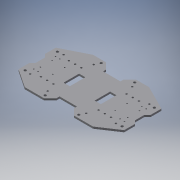
# Autodesk Inventor part: Support_Moteur
Saved by Autodesk Inventor 2016 (Build 200138000, 138)
## iProperties
Created: 2015-09-29
Part Number: Support_Moteur
Material: Générique
Document SubType Name: Modeling
Designer: Logan
Density: 1 g/cm^3
Appearance: Par défaut
Author: Logan
Autodesk Inventor part; units mm, degrees
ref_plane "YZ Plane" through (0, 0, 0) normal (1, 0, 0) x (0, 1, 0)
ref_plane "XZ Plane" through (0, 0, 0) normal (0, 1, 0) x (-1, 0, 0)
ref_plane "XY Plane" through (0, 0, 0) normal (0, 0, 1) x (1, 0, 0)
sketch "Esquisse1" plane through (0, 0, 0) normal (0, 0, 1) x (1, 0, 0)
  line L0 (-170, -60) -> (-170, 60)
  line L1 (170, 60) -> (170, -60)
  line L2 (170, -100) -> (-170, 100) construction
  line L3 (-170, -100) -> (170, 100) construction
  line L4 (-90, 100) -> (-170, 60)
  line L5 (90, 100) -> (170, 60)
  line L6 (-170, -60) -> (-110, -100)
  line L7 (110, -100) -> (170, -60)
  line L8 (48, 100) -> (90, 100)
  line L9 (52, 0) -> (-69, 0)
  line L10 (28, -80) -> (28, -70)
  line L11 (28, -70) -> (-28, -70)
  line L12 (-28, -70) -> (-28, -80)
  line L13 (-28, -80) -> (-48, -100)
  line L14 (28, -80) -> (48, -100)
  line L15 (110, -100) -> (48, -100)
  line L16 (-48, -100) -> (-110, -100)
  line L17 (-28, 70) -> (-28, 80)
  line L18 (-28, 80) -> (-48, 100)
  line L19 (28, 70) -> (-28, 70)
  line L20 (28, 80) -> (28, 70)
  line L21 (28, 80) -> (48, 100)
  line L22 (-90, 100) -> (-48, 100)
  line L23 (48, 100) -> (90, 100)
  point P0 (0, 0)
  dimension "d2" = 80
  dimension "d3" = 40
  dimension "d4" = 80
  dimension "d5" = 40
  dimension "d6" = 40
  dimension "d7" = 60
  dimension "d8" = 60
  dimension "d9" = 40
  constraints: 48 end point, 7 parallel, 6 symmetric about line, 4 point on line, 3 horizontal, 2 collinear, 2 midpoint, 2 perpendicular
  measures "d2" distance of L4.start L2.end
  measures "d3" distance of L0.end L2.end
  measures "d4" distance of L5.start L3.end
  measures "d5" distance of L1.start L3.end
  measures "d6" distance of L0.start L3.start
  measures "d7" distance of L6.end L3.start
  measures "d8" distance of L7.start L2.start
  measures "d9" distance of L1.end L2.start
extrude "Plaque" add sketch "Esquisse1" along normal blind 6
sketch "Esquisse2" plane through (0, 0, 6) normal (0, 0, 1) x (1, 0, 0)
  circle A0 centre (-146, 35) radius 2
  circle A1 centre (-132, 35) radius 2
  circle A2 centre (-146, -35) radius 2
  circle A3 centre (-132, -35) radius 2
  line L0 (-170, 60) -> (-170, -60) projected
  line L1 (0, 25.5561) -> (0, -26.1527)
  circle A4 centre (146, 35) radius 2
  circle A5 centre (132, 35) radius 2
  circle A6 centre (146, -35) radius 2
  circle A7 centre (132, -35) radius 2
  point P0 (0, 0)
  dimension "d12" = 4
  dimension "d13" = 4
  dimension "d14" = 4
  dimension "d15" = 4
  dimension "d16" = 14
  dimension "d17" = 14
  dimension "d18" = 24
  dimension "d19" = 24
  dimension "d20" = 35
  dimension "d21" = 35
  dimension "d22" = 35
  dimension "d23" = 35
  constraints: 8 centre point, 4 symmetric about line, 2 end point, 1 vertical, 4 other
  measures "d12" diameter of A0
  measures "d13" diameter of A1
  measures "d14" diameter of A3
  measures "d15" diameter of A2
  measures "d16" distance of A1.centre A0.centre
  measures "d17" distance of A3.centre A2.centre
  measures "d18" distance from line of L0 A0.centre
  measures "d19" distance from line of L0 A2.centre
  measures "d20" vertical distance of point (0, 0) A2.centre
  measures "d21" vertical distance of point (0, 0) A3.centre
  measures "d22" vertical distance of point (0, 0) A1.centre
  measures "d23" vertical distance of point (0, 0) A0.centre
hole "Fixation_Encodeur" at (-132, 35, 6) at (-146, 35, 6) at (-146, -35, 6) at (-132, -35, 6) at (132, 35, 6) at (146, 35, 6) at (146, -35, 6) at (132, -35, 6) direction (0, 0, -1) diameter 4 end through all
sketch "Esquisse3" plane through (0, 0, 6) normal (0, 0, 1) x (1, 0, 0)
  line L0 (-140.5, -19) -> (-100.5, -19)
  line L1 (-100.5, -19) -> (-100.5, 19)
  line L2 (-100.5, 19) -> (-140.5, 19)
  line L3 (-140.5, 19) -> (-140.5, -19)
  line L4 (-140.5, -19) -> (-100.5, 19) construction
  line L5 (-100.5, -19) -> (-140.5, 19) construction
  line L6 (-90, 100) -> (-170, 60) projected
  line L7 (-170, 60) -> (-170, -60) projected
  line L8 (-170, -60) -> (-110, -100) projected
  line L9 (48, -100) -> (110, -100) projected
  line L10 (110, -100) -> (170, -60) projected
  line L11 (170, -60) -> (170, 60) projected
  line L12 (170, 60) -> (90, 100) projected
  line L13 (-48, 100) -> (-90, 100) projected
  line L14 (0, 102.1518) -> (0, -90)
  line L15 (140.5, -19) -> (100.5, -19)
  line L16 (100.5, -19) -> (100.5, 19)
  line L17 (100.5, 19) -> (140.5, 19)
  line L18 (140.5, 19) -> (140.5, -19)
  line L19 (140.5, -19) -> (100.5, 19) construction
  line L20 (100.5, -19) -> (140.5, 19) construction
  line L21 (-110, -100) -> (-48, -100) projected
  line L22 (-48, -100) -> (-28, -80) projected
  line L23 (-28, -80) -> (-28, -70) projected
  line L24 (-28, -70) -> (28, -70) projected
  line L25 (28, -70) -> (28, -80) projected
  line L26 (28, -80) -> (48, -100) projected
  line L27 (90, 100) -> (48, 100) projected
  line L28 (48, 100) -> (28, 80) projected
  line L29 (28, 80) -> (28, 70) projected
  line L30 (28, 70) -> (-28, 70) projected
  line L31 (-28, 70) -> (-28, 80) projected
  line L32 (-28, 80) -> (-48, 100) projected
  point P0 (0, 0)
  point P1 (-120.5, 0)
  point P2 (120.5, 0)
  dimension "d31" = 29.5
  dimension "d32" = 40
  dimension "d33" = 38
  dimension "d53" = 19
  constraints: 26 end point, 5 symmetric about line, 4 midpoint, 2 parallel, 1 horizontal, 1 perpendicular, 1 vertical
  measures "d31" distance between parallel lines of L7 L3
  measures "d32" distance between parallel lines of L3 L1
  measures "d33" distance between parallel lines of L0 L2
  measures "d53" distance from line of point (0, 0) L2
hole "Fixation_Moteur" at (-140.5, 19, 6) at (-100.5, 19, 6) at (-100.5, -19, 6) at (-140.5, -19, 6) at (140.5, 19, 6) at (140.5, -19, 6) at (100.5, 19, 6) at (100.5, -19, 6) direction (0, 0, -1) diameter 4 end through all
sketch "Esquisse4" plane through (0, 0, 6) normal (0, 0, 1) x (1, 0, 0)
  line L0 (-60, -25) -> (-40, -25)
  line L1 (-60, 25) -> (-60, -25)
  line L2 (-60, -25) -> (-39.915, 7.067) construction
  circle A0 centre (100.5, 19) radius 2 projected
  circle A1 centre (140.5, 19) radius 2 projected
  circle A2 centre (-100.5, -19) radius 2 projected
  circle A3 centre (-140.5, 19) radius 2 projected
  circle A4 centre (-100.5, 19) radius 2 projected
  circle A5 centre (-140.5, -19) radius 2 projected
  circle A6 centre (140.5, -19) radius 2 projected
  circle A7 centre (100.5, -19) radius 2 projected
  line L3 (-90, 100) -> (-170, 60) projected
  line L4 (-170, 60) -> (-170, -60) projected
  line L5 (-170, -60) -> (-110, -100) projected
  line L6 (48, -100) -> (110, -100) projected
  line L7 (110, -100) -> (170, -60) projected
  line L8 (170, -60) -> (170, 60) projected
  line L9 (170, 60) -> (90, 100) projected
  line L10 (-48, 100) -> (-90, 100) projected
  line L11 (40, 25) -> (60, 25)
  line L12 (60, 25) -> (60, -25)
  line L13 (60, -25) -> (40, -10.6364) construction
  line L14 (40, 25) -> (40, -25)
  line L15 (-40, -25) -> (-40, 25)
  line L16 (-40, 25) -> (-60, 25)
  line L17 (-39.915, 7.067) -> (-60, 25) construction
  line L18 (40, 10.0232) -> (60, 25) construction
  line L19 (60, -25) -> (40, -25)
  line L20 (-110, -100) -> (-48, -100) projected
  line L21 (-48, -100) -> (-28, -80) projected
  line L22 (-28, -80) -> (-28, -70) projected
  line L23 (-28, -70) -> (28, -70) projected
  line L24 (28, -70) -> (28, -80) projected
  line L25 (28, -80) -> (48, -100) projected
  line L26 (90, 100) -> (48, 100) projected
  line L27 (48, 100) -> (28, 80) projected
  line L28 (28, 80) -> (28, 70) projected
  line L29 (28, 70) -> (-28, 70) projected
  line L30 (-28, 70) -> (-28, 80) projected
  line L31 (-28, 80) -> (-48, 100) projected
  point P0 (-39.915, 7.067)
  dimension "d50" = 110
  dimension "d157" = 110
  dimension "d158" = 20
  dimension "d159" = 20
  constraints: 24 end point, 3 point on line, 2 collinear, 2 parallel, 1 horizontal
  measures "d50" distance between parallel lines of L4 L1
  measures "d157" distance between parallel lines of L8 L12
  measures "d158" distance between parallel lines of L1 L15
  measures "d159" distance between parallel lines of L12 L14
extrude "Passage_Courroie" cut sketch "Esquisse4" against normal up to surface (6 mm away) contours L1 L16 L15 L0 | L11 L12 L19 L14
sketch "Esquisse5" plane through (0, 0, 6) normal (0, 0, 1) x (1, 0, 0)
  line L0 (0, 30.4597) -> (0, -30.4597)
  line L1 (-17.5456, 0) -> (17.5456, 0)
  line L2 (-80, 40) -> (-80, -40)
  line L3 (-80, -40) -> (-110, -40)
  line L4 (-110, 30) -> (-110, 40)
  line L5 (-110, 40) -> (-80, 40)
  line L6 (-88, 90) -> (-142, 63)
  line L7 (-142, 63) -> (-142, 30)
  line L8 (-142, 30) -> (-110, 30)
  line L9 (-110, -30) -> (-142, -30)
  line L10 (-142, -30) -> (-142, -63)
  line L11 (-142, -63) -> (-102, -90)
  line L12 (-102, -90) -> (-44, -90)
  line L13 (-44, -90) -> (-34, -80)
  line L14 (-34, -80) -> (-34, 80)
  line L15 (-34, 80) -> (-44, 90)
  line L16 (-44, 90) -> (-88, 90)
  line L17 (-110, -40) -> (-110, -30)
  circle A0 centre (-134, -35) radius 2
  circle A1 centre (-134, 35) radius 2
  circle A2 centre (-120, 35) radius 2
  circle A3 centre (-120, -35) radius 2
  line L18 (-88, 90) -> (-142, 63)
  line L19 (-142, 63) -> (-142, 30)
  line L20 (-142, 30) -> (-110, 30)
  line L21 (-110, 30) -> (-110, 40)
  line L22 (-110, 40) -> (-80, 40)
  line L23 (-80, 40) -> (-80, -40)
  line L24 (-80, -40) -> (-110, -40)
  line L25 (-110, -40) -> (-110, -30)
  line L26 (-110, -30) -> (-142, -30)
  line L27 (-142, -30) -> (-142, -63)
  line L28 (-142, -63) -> (-102, -90)
  line L29 (-102, -90) -> (-44, -90)
  line L30 (-44, -90) -> (-34, -80)
  line L31 (-34, -80) -> (-34, 80)
  line L32 (-34, 80) -> (-44, 90)
  line L33 (-44, 90) -> (-88, 90)
  line L34 (-138, 53.1115) -> (-96.2229, 74)
  line L35 (-96.2229, 74) -> (-62, 74)
  line L36 (-62, 74) -> (-62, -74)
  line L37 (-62, -74) -> (-109.1054, -74)
  line L38 (-109.1054, -74) -> (-138, -54.4961)
  line L39 (96.2229, 74) -> (62, 74)
  line L40 (138, 53.1115) -> (96.2229, 74)
  line L41 (62, -74) -> (109.1054, -74)
  line L42 (109.1054, -74) -> (138, -54.4961)
  line L43 (-170, 60) -> (-170, -60) projected
  point P0 (0, 0)
  point P1 (72.8, -45)
  point P2 (92.8, -45)
  point P3 (112.8, -45)
  point P4 (-72.8, -45)
  point P5 (-92.8, -45)
  point P6 (-112.8, -45)
  point P7 (72.8, 45)
  point P8 (92.8, 45)
  point P9 (112.8, 45)
  point P10 (-72.8, 45)
  point P11 (-92.8, 45)
  point P12 (-112.8, 45)
  point P13 (0, 0)
  dimension "d14" = 4
  dimension "d174" = 10.6334
  dimension "d175" = 47.1054
  dimension "d176" = 34.2229
  dimension "d177" = 41.7771
  dimension "d178" = 28.8946
  dimension "d179" = 32
  dimension "d180" = 32
  constraints: 86 end point, 15 symmetric about line, 4 centre point, 2 midpoint, 2 vertical, 1 coincident, 1 horizontal
  measures "d174" distance between parallel lines of L6 L34
  measures "d175" distance of L36.end L37.end
  measures "d176" distance of L35.start L35.end
  measures "d177" horizontal distance of L34.start L35.start
  measures "d178" horizontal distance of L37.end L38.end
  measures "d179" distance from line of L43 L38.end
  measures "d180" distance from line of L43 L34.start
hole "Fixation_Base" at (72.8, -45, 6) at (92.8, -45, 6) at (112.8, -45, 6) at (-112.8, 45, 6) at (-72.8, 45, 6) at (-92.8, 45, 6) at (-112.8, -45, 6) at (-92.8, -45, 6) at (-72.8, -45, 6) at (72.8, 45, 6) at (92.8, 45, 6) at (112.8, 45, 6) at (138, 53.1115, 6) at (62, 74, 6) at (138, -54.4961, 6) at (62, -74, 6) at (-62, -74, 6) at (-138, -54.4961, 6) at (-138, 53.1115, 6) at (-62, 74, 6) direction (0, 0, -1) diameter 6 end through all
sketch "Esquisse7" plane through (0, 0, 6) normal (0, 0, 1) x (1, 0, 0)
  line L0 (-54, 90) -> (54, 90)
  line L1 (-156, 0) -> (156, 0)
  line L2 (-170, 60) -> (-170, -60) projected
  line L3 (170, -60) -> (170, 60) projected
  line L4 (-110, -100) -> (110, -100) projected
  line L5 (-48, 100) -> (-90, 100) projected
  line L6 (-156, 0) -> (-156, 51.3475)
  line L7 (-156, 0) -> (-156, -52.5074)
  line L8 (156, 0) -> (156, 51.3475)
  line L9 (156, 0) -> (156, -52.5074)
  line L10 (-90, 100) -> (-170, 60) projected
  line L11 (170, 60) -> (90, 100) projected
  line L12 (110, -100) -> (170, -60) projected
  line L13 (-170, -60) -> (-110, -100) projected
  point P0 (0, 0)
  point P1 (-54, -90)
  point P2 (54, -90)
  dimension "d88" = 14
  dimension "d89" = 14
  dimension "d93" = 10
  dimension "d94" = 108
  dimension "d95" = 54
  dimension "d123" = 108
  dimension "d124" = 10
  dimension "d125" = 10
  dimension "d126" = 56
  dimension "d160" = 56
  dimension "d181" = 14
  dimension "d182" = 14
  dimension "d186" = 14
  dimension "d187" = 14
  constraints: 12 end point, 4 vertical, 3 horizontal
  measures "d88" distance from line of L2 L1.start
  measures "d89" distance from line of L3 L1.end
  measures "d93" distance between parallel lines of L0 L5
  measures "d94" distance of L0.start L0.end
  measures "d95" horizontal distance of point (0, 0) L0.start
  measures "d123" distance of point (54, -90) point (-54, -90)
  measures "d124" distance from line of L4 point (54, -90)
  measures "d125" distance from line of L4 point (-54, -90)
  measures "d126" horizontal distance of L4.start point (-54, -90)
  measures "d160" horizontal distance of L4.end point (54, -90)
  measures "d181" distance from line of L10 L6.end
  measures "d182" distance from line of L11 L8.end
  measures "d186" distance from line of L12 L9.end
  measures "d187" distance from line of L13 L7.end
hole "Fixation_Etage3" at (-54, 90, 6) at (-54, -90, 6) at (54, -90, 6) at (54, 90, 6) at (-156, 51.3475, 6) at (-156, -52.5074, 6) at (156, 51.3475, 6) at (156, -52.5074, 6) direction (0, 0, -1) diameter 8 end through all
sketch "Esquisse8" plane through (0, 0, 6) normal (0, 0, 1) x (1, 0, 0)
  line L0 (-160, -25) -> (-170, -25)
  line L1 (-170, -25) -> (-170, 25)
  line L2 (-170, 25) -> (-160, 25)
  line L3 (-160, 25) -> (-160, -25)
  line L4 (-160, -25) -> (-170, 25) construction
  line L5 (-170, -25) -> (-160, 25) construction
  line L6 (0, 43.7993) -> (0, -83.0015)
  line L7 (160, -25) -> (170, -25)
  line L8 (170, -25) -> (170, 25)
  line L9 (170, 25) -> (160, 25)
  line L10 (160, 25) -> (160, -25)
  line L11 (160, -25) -> (170, 25) construction
  line L12 (170, -25) -> (160, 25) construction
  point P0 (0, 0)
  point P1 (-165, 0)
  point P2 (165, 0)
  dimension "d106" = 50
  dimension "d107" = 10
  dimension "d108" = 160
  dimension "d191" = 25
  constraints: 26 end point, 5 symmetric about line, 4 midpoint, 2 parallel, 1 horizontal, 1 perpendicular, 1 vertical
  measures "d106" distance of L2.end L0.start
  measures "d107" distance of L1.end L2.end
  measures "d108" distance from line of point (0, 0) L3
  measures "d191" distance from line of point (0, 0) L2
extrude "Passage_Encodeur" cut sketch "Esquisse8" against normal up to surface (6 mm away)
chamfer "Chanfrein1" distance 10 angle 45 4 edges at (-160, 25, 3) (-160, -25, 3) (160, 25, 3) (160, -25, 3)
